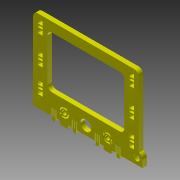
# Autodesk Inventor part: front
Saved by Autodesk Inventor 2012 SP1 (Build 160190100, 190)
## iProperties
Created: 2011-10-14
Part Number: front
Document SubType Name: Modeling
Designer: cramera
Density: 0.952 g/cm^3
Material: High Density Polyethylene
Mass: 331.479 g
Surface Area: 1014.12 cm^2
Volume: 348.192 cm^3
Autodesk Inventor part; units mm, degrees
ref_plane "YZ Plane" through (0, 0, 0) normal (1, 0, 0) x (0, 1, 0)
ref_plane "XZ Plane" through (0, 0, 0) normal (0, 1, 0) x (-1, 0, 0)
ref_plane "XY Plane" through (0, 0, 0) normal (0, 0, 1) x (1, 0, 0)
derived "skeleton.ipt"
sketch "DRILL-THROUGH" plane through (0, 0, 0) normal (0, 0, 1) x (1, 0, 0)
  arc A0 (646.0554, 82.7451) -> (647.6429, 84.3326) centre (646.0554, 84.3326) ccw
  arc A1 (646.0554, 116.9081) -> (644.4679, 115.3206) centre (646.0554, 115.3206) ccw
  arc A2 (644.4679, 115.3206) -> (646.0554, 113.7331) centre (646.0554, 115.3206) ccw
  arc A3 (646.0554, 113.7331) -> (647.6429, 115.3206) centre (646.0554, 115.3206) ccw
  arc A4 (647.6429, 115.3206) -> (646.0554, 116.9081) centre (646.0554, 115.3206) ccw
  arc A5 (677.0434, 116.9081) -> (675.4559, 115.3206) centre (677.0434, 115.3206) ccw
  arc A6 (675.4559, 115.3206) -> (677.0434, 113.7331) centre (677.0434, 115.3206) ccw
  arc A7 (677.0434, 113.7331) -> (678.6309, 115.3206) centre (677.0434, 115.3206) ccw
  arc A8 (678.6309, 115.3206) -> (677.0434, 116.9081) centre (677.0434, 115.3206) ccw
  arc A9 (646.0554, 85.9201) -> (644.4679, 84.3326) centre (646.0554, 84.3326) ccw
  arc A10 (644.4679, 84.3326) -> (646.0554, 82.7451) centre (646.0554, 84.3326) ccw
  arc A11 (647.6429, 84.3326) -> (646.0554, 85.9201) centre (646.0554, 84.3326) ccw
  arc A12 (677.0434, 85.9201) -> (675.4559, 84.3326) centre (677.0434, 84.3326) ccw
  arc A13 (675.4559, 84.3326) -> (677.0434, 82.7451) centre (677.0434, 84.3326) ccw
  arc A14 (677.0434, 82.7451) -> (678.6309, 84.3326) centre (677.0434, 84.3326) ccw
  arc A15 (678.6309, 84.3326) -> (677.0434, 85.9201) centre (677.0434, 84.3326) ccw
  constraints: 32 point on circle, 16 centre point
sketch "POCKET_1-16" plane through (0, 0, 0) normal (0, 0, 1) x (1, 0, 0)
  line L0 (766.5149, 230.5307) -> (766.5149, 224.7099)
  arc A0 (766.5149, 224.7099) -> (768.1024, 223.1224) centre (768.1024, 224.7099) ccw
  line L1 (768.1024, 223.1224) -> (774.717, 223.1224)
  arc A1 (774.717, 223.1224) -> (776.3045, 224.7099) centre (774.717, 224.7099) ccw
  line L2 (776.3045, 224.7099) -> (776.3045, 230.5307)
  arc A2 (776.3045, 230.5307) -> (774.717, 232.1182) centre (774.717, 230.5307) ccw
  arc A3 (776.3045, 238.6005) -> (771.4097, 243.4953) centre (771.4097, 238.6005) ccw
  arc A4 (771.4097, 243.4953) -> (766.5149, 238.6005) centre (771.4097, 238.6005) ccw
  arc A5 (766.5149, 238.6005) -> (771.4097, 233.7057) centre (771.4097, 238.6005) ccw
  arc A6 (771.4097, 233.7057) -> (776.3045, 238.6005) centre (771.4097, 238.6005) ccw
  line L3 (774.717, 232.1182) -> (768.1024, 232.1182)
  arc A7 (790.0628, 221.5349) -> (788.4753, 219.9474) centre (790.0628, 219.9474) ccw
  line L4 (788.4753, 219.9474) -> (788.4753, 213.3328)
  arc A8 (788.4753, 213.3328) -> (790.0628, 211.7453) centre (790.0628, 213.3328) ccw
  line L5 (790.0628, 211.7453) -> (796.6774, 211.7453)
  arc A9 (796.6774, 211.7453) -> (798.2649, 213.3328) centre (796.6774, 213.3328) ccw
  line L6 (798.2649, 213.3328) -> (798.2649, 219.9474)
  arc A10 (798.2649, 219.9474) -> (796.6774, 221.5349) centre (796.6774, 219.9474) ccw
  line L7 (796.6774, 221.5349) -> (790.0628, 221.5349)
  arc A11 (768.1024, 221.5349) -> (766.5149, 219.9474) centre (768.1024, 219.9474) ccw
  line L8 (766.5149, 219.9474) -> (766.5149, 213.3328)
  arc A12 (766.5149, 213.3328) -> (768.1024, 211.7453) centre (768.1024, 213.3328) ccw
  line L9 (768.1024, 211.7453) -> (774.717, 211.7453)
  arc A13 (774.717, 211.7453) -> (776.3045, 213.3328) centre (774.717, 213.3328) ccw
  line L10 (776.3045, 213.3328) -> (776.3045, 219.9474)
  arc A14 (776.3045, 219.9474) -> (774.717, 221.5349) centre (774.717, 219.9474) ccw
  line L11 (774.717, 221.5349) -> (768.1024, 221.5349)
  arc A15 (785.3003, 233.7057) -> (786.8878, 235.2932) centre (785.3003, 235.2932) ccw
  line L12 (786.8878, 235.2932) -> (786.8878, 241.9078)
  arc A16 (786.8878, 241.9078) -> (785.3003, 243.4953) centre (785.3003, 241.9078) ccw
  line L13 (785.3003, 243.4953) -> (779.4795, 243.4953)
  arc A17 (779.4795, 243.4953) -> (777.892, 241.9078) centre (779.4795, 241.9078) ccw
  line L14 (777.892, 241.9078) -> (777.892, 235.2932)
  arc A18 (777.892, 235.2932) -> (779.4795, 233.7057) centre (779.4795, 235.2932) ccw
  line L15 (779.4795, 233.7057) -> (785.3003, 233.7057)
  arc A19 (790.0628, 232.1182) -> (788.4753, 230.5307) centre (790.0628, 230.5307) ccw
  line L16 (788.4753, 230.5307) -> (788.4753, 224.7099)
  arc A20 (788.4753, 224.7099) -> (790.0628, 223.1224) centre (790.0628, 224.7099) ccw
  line L17 (790.0628, 223.1224) -> (796.6774, 223.1224)
  line L18 (798.2649, 224.7099) -> (798.2649, 230.5307)
  arc A21 (798.2649, 230.5307) -> (796.6774, 232.1182) centre (796.6774, 230.5307) ccw
  line L19 (796.6774, 232.1182) -> (790.0628, 232.1182)
  arc A22 (796.6774, 223.1224) -> (798.2649, 224.7099) centre (796.6774, 224.7099) ccw
  line L20 (777.892, 219.9474) -> (777.892, 213.3328)
  arc A23 (777.892, 213.3328) -> (779.4795, 211.7453) centre (779.4795, 213.3328) ccw
  line L21 (779.4795, 211.7453) -> (785.3003, 211.7453)
  arc A24 (785.3003, 211.7453) -> (786.8878, 213.3328) centre (785.3003, 213.3328) ccw
  line L22 (786.8878, 213.3328) -> (786.8878, 219.9474)
  arc A25 (786.8878, 219.9474) -> (785.3003, 221.5349) centre (785.3003, 219.9474) ccw
  line L23 (785.3003, 221.5349) -> (779.4795, 221.5349)
  arc A26 (786.8878, 227.6203) -> (782.3899, 232.1182) centre (782.3899, 227.6203) ccw
  arc A27 (782.3899, 232.1182) -> (777.892, 227.6203) centre (782.3899, 227.6203) ccw
  arc A28 (788.4753, 235.2932) -> (790.0628, 233.7057) centre (790.0628, 235.2932) ccw
  line L24 (790.0628, 233.7057) -> (796.6774, 233.7057)
  arc A29 (779.4795, 221.5349) -> (777.892, 219.9474) centre (779.4795, 219.9474) ccw
  arc A30 (768.1024, 232.1182) -> (766.5149, 230.5307) centre (768.1024, 230.5307) ccw
  arc A31 (777.892, 227.6203) -> (782.3899, 223.1224) centre (782.3899, 227.6203) ccw
  arc A32 (782.3899, 223.1224) -> (786.8878, 227.6203) centre (782.3899, 227.6203) ccw
  arc A33 (796.6774, 233.7057) -> (798.2649, 235.2932) centre (796.6774, 235.2932) ccw
  line L25 (798.2649, 235.2932) -> (798.2649, 241.9078)
  arc A34 (798.2649, 241.9078) -> (796.6774, 243.4953) centre (796.6774, 241.9078) ccw
  line L26 (796.6774, 243.4953) -> (790.0628, 243.4953)
  arc A35 (790.0628, 243.4953) -> (788.4753, 241.9078) centre (790.0628, 241.9078) ccw
  line L27 (788.4753, 241.9078) -> (788.4753, 235.2932)
  constraints: 72 point on circle, 56 end point, 36 centre point
sketch "POCKET_3-8" plane through (0, 0, 0) normal (0, 0, 1) x (1, 0, 0)
  circle A0 centre (796.1694, 92.6193) radius 12.7
  constraints: 1 centre point
sketch "STOCK_12MM" plane through (0, 0, 0) normal (0, 0, 1) x (1, 0, 0)
  line L0 (457.2, 0) -> (914.4, 0)
  line L1 (914.4, 0) -> (914.4, 914.4)
  line L2 (914.4, 914.4) -> (457.2, 914.4)
  line L3 (457.2, 914.4) -> (457.2, 0)
  line L4 (457.2, 0) -> (457.2, 914.4)
  constraints: 10 end point
sketch "THROUGH-CUT" plane through (0, 0, 0) normal (0, 0, 1) x (1, 0, 0)
  line L0 (546.8684, 124.1379) -> (546.8684, 124.7278)
  arc A0 (546.8684, 124.7278) -> (546.8684, 126.9728) centre (545.7459, 125.8503) ccw
  arc A1 (546.8684, 126.9728) -> (544.6234, 126.9728) centre (545.7459, 125.8503) ccw
  line L1 (544.6234, 126.9728) -> (536.7945, 126.9728)
  circle A2 centre (604.3994, 99.8266) radius 5.925
  circle A3 centre (718.6994, 99.8266) radius 5.925
  circle A4 centre (796.1694, 92.6193) radius 7.3025
  circle A5 centre (661.5494, 99.8266) radius 14.2875
  line L2 (534.5494, 116.3458) -> (534.5494, 110.6759)
  arc A6 (534.5494, 110.6759) -> (534.5494, 108.4308) centre (535.6719, 109.5534) ccw
  arc A7 (534.5494, 108.4308) -> (536.7945, 108.4308) centre (535.6719, 109.5534) ccw
  line L3 (536.7945, 108.4308) -> (544.6234, 108.4308)
  arc A8 (544.6234, 108.4308) -> (546.8684, 110.6759) centre (545.7459, 109.5534) ccw
  line L4 (546.8684, 110.6759) -> (546.8684, 116.3458)
  arc A9 (546.8684, 116.3458) -> (546.8684, 118.5908) centre (545.7459, 117.4683) ccw
  arc A10 (546.8684, 118.5908) -> (544.6234, 118.5908) centre (545.7459, 117.4683) ccw
  line L5 (544.6234, 118.5908) -> (536.7945, 118.5908)
  arc A11 (536.7945, 118.5908) -> (534.5494, 116.3458) centre (535.6719, 117.4683) ccw
  line L6 (536.7945, 130.2748) -> (544.6234, 130.2748)
  arc A12 (544.6234, 130.2748) -> (546.8684, 130.2748) centre (545.7459, 131.3974) ccw
  arc A13 (546.8684, 130.2748) -> (546.8684, 132.5199) centre (545.7459, 131.3974) ccw
  line L7 (546.8684, 132.5199) -> (546.8684, 138.1898)
  arc A14 (546.8684, 138.1898) -> (546.8684, 140.4348) centre (545.7459, 139.3123) ccw
  arc A15 (546.8684, 140.4348) -> (544.6234, 140.4348) centre (545.7459, 139.3123) ccw
  line L8 (544.6234, 140.4348) -> (536.7945, 140.4348)
  arc A16 (536.7945, 140.4348) -> (534.5494, 138.1898) centre (535.6719, 139.3123) ccw
  line L9 (534.5494, 138.1898) -> (534.5494, 132.5199)
  arc A17 (534.5494, 132.5199) -> (536.7945, 130.2748) centre (535.6719, 131.3974) ccw
  line L10 (534.5494, 256.0458) -> (534.5494, 250.3759)
  arc A18 (534.5494, 250.3759) -> (534.5494, 248.1308) centre (535.6719, 249.2534) ccw
  arc A19 (534.5494, 248.1308) -> (536.7945, 248.1308) centre (535.6719, 249.2534) ccw
  line L11 (536.7945, 248.1308) -> (544.6234, 248.1308)
  arc A20 (544.6234, 248.1308) -> (546.8684, 248.1308) centre (545.7459, 249.2534) ccw
  arc A21 (546.8684, 248.1308) -> (546.8684, 250.3759) centre (545.7459, 249.2534) ccw
  line L12 (546.8684, 250.3759) -> (546.8684, 256.0458)
  arc A22 (546.8684, 256.0458) -> (546.8684, 258.2908) centre (545.7459, 257.1683) ccw
  arc A23 (546.8684, 258.2908) -> (544.6234, 258.2908) centre (545.7459, 257.1683) ccw
  line L13 (544.6234, 258.2908) -> (536.7945, 258.2908)
  arc A24 (536.7945, 258.2908) -> (534.5494, 258.2908) centre (535.6719, 257.1683) ccw
  arc A25 (534.5494, 258.2908) -> (534.5494, 256.0458) centre (535.6719, 257.1683) ccw
  arc A26 (786.3044, 248.1308) -> (788.5494, 250.3759) centre (787.4269, 249.2534) ccw
  line L14 (788.5494, 250.3759) -> (788.5494, 256.0458)
  arc A27 (788.5494, 256.0458) -> (786.3044, 258.2908) centre (787.4269, 257.1683) ccw
  line L15 (786.3044, 258.2908) -> (778.4755, 258.2908)
  arc A28 (778.4755, 258.2908) -> (776.2304, 256.0458) centre (777.3529, 257.1683) ccw
  line L16 (776.2304, 256.0458) -> (776.2304, 250.3759)
  arc A29 (776.2304, 250.3759) -> (778.4755, 248.1308) centre (777.3529, 249.2534) ccw
  line L17 (778.4755, 248.1308) -> (786.3044, 248.1308)
  arc A30 (786.3044, 269.9748) -> (788.5494, 272.2199) centre (787.4269, 271.0974) ccw
  line L18 (788.5494, 272.2199) -> (788.5494, 277.8898)
  arc A31 (788.5494, 277.8898) -> (786.3044, 280.1348) centre (787.4269, 279.0123) ccw
  line L19 (786.3044, 280.1348) -> (778.4755, 280.1348)
  arc A32 (778.4755, 280.1348) -> (776.2304, 277.8898) centre (777.3529, 279.0123) ccw
  line L20 (776.2304, 277.8898) -> (776.2304, 272.2199)
  arc A33 (776.2304, 272.2199) -> (778.4755, 269.9748) centre (777.3529, 271.0974) ccw
  line L21 (778.4755, 269.9748) -> (786.3044, 269.9748)
  arc A34 (536.7945, 193.6478) -> (534.5494, 191.4028) centre (535.6719, 192.5253) ccw
  line L22 (534.5494, 191.4028) -> (534.5494, 190.8129)
  arc A35 (534.5494, 190.8129) -> (536.7945, 188.5678) centre (535.6719, 189.6904) ccw
  line L23 (536.7945, 188.5678) -> (544.6234, 188.5678)
  arc A36 (544.6234, 188.5678) -> (546.8684, 188.5678) centre (545.7459, 189.6904) ccw
  arc A37 (546.8684, 188.5678) -> (546.8684, 190.8129) centre (545.7459, 189.6904) ccw
  line L24 (546.8684, 190.8129) -> (546.8684, 191.4028)
  arc A38 (546.8684, 191.4028) -> (546.8684, 193.6478) centre (545.7459, 192.5253) ccw
  arc A39 (546.8684, 193.6478) -> (544.6234, 193.6478) centre (545.7459, 192.5253) ccw
  line L25 (544.6234, 193.6478) -> (536.7945, 193.6478)
  arc A40 (786.3044, 261.5928) -> (788.5494, 263.8379) centre (787.4269, 262.7154) ccw
  line L26 (788.5494, 263.8379) -> (788.5494, 264.4278)
  arc A41 (788.5494, 264.4278) -> (786.3044, 266.6728) centre (787.4269, 265.5503) ccw
  line L27 (786.3044, 266.6728) -> (778.4755, 266.6728)
  arc A42 (778.4755, 266.6728) -> (776.2304, 264.4278) centre (777.3529, 265.5503) ccw
  line L28 (776.2304, 264.4278) -> (776.2304, 263.8379)
  arc A43 (776.2304, 263.8379) -> (778.4755, 261.5928) centre (777.3529, 262.7154) ccw
  line L29 (778.4755, 261.5928) -> (786.3044, 261.5928)
  line L30 (534.5494, 204.8648) -> (534.5494, 199.1949)
  arc A44 (534.5494, 199.1949) -> (534.5494, 196.9498) centre (535.6719, 198.0724) ccw
  arc A45 (534.5494, 196.9498) -> (536.7945, 196.9498) centre (535.6719, 198.0724) ccw
  line L31 (536.7945, 196.9498) -> (544.6234, 196.9498)
  arc A46 (544.6234, 196.9498) -> (546.8684, 196.9498) centre (545.7459, 198.0724) ccw
  arc A47 (546.8684, 196.9498) -> (546.8684, 199.1949) centre (545.7459, 198.0724) ccw
  line L32 (546.8684, 199.1949) -> (546.8684, 204.8648)
  arc A48 (546.8684, 204.8648) -> (546.8684, 207.1098) centre (545.7459, 205.9873) ccw
  arc A49 (546.8684, 207.1098) -> (544.6234, 207.1098) centre (545.7459, 205.9873) ccw
  line L33 (544.6234, 207.1098) -> (536.7945, 207.1098)
  arc A50 (536.7945, 207.1098) -> (534.5494, 204.8648) centre (535.6719, 205.9873) ccw
  line L34 (534.5494, 183.0208) -> (534.5494, 177.3509)
  arc A51 (534.5494, 177.3509) -> (534.5494, 175.1058) centre (535.6719, 176.2284) ccw
  arc A52 (534.5494, 175.1058) -> (536.7945, 175.1058) centre (535.6719, 176.2284) ccw
  line L35 (536.7945, 175.1058) -> (544.6234, 175.1058)
  arc A53 (544.6234, 175.1058) -> (546.8684, 177.3509) centre (545.7459, 176.2284) ccw
  line L36 (546.8684, 177.3509) -> (546.8684, 183.0208)
  arc A54 (546.8684, 183.0208) -> (546.8684, 185.2658) centre (545.7459, 184.1433) ccw
  arc A55 (546.8684, 185.2658) -> (544.6234, 185.2658) centre (545.7459, 184.1433) ccw
  line L37 (544.6234, 185.2658) -> (536.7945, 185.2658)
  arc A56 (536.7945, 185.2658) -> (534.5494, 183.0208) centre (535.6719, 184.1433) ccw
  arc A57 (786.3044, 175.1058) -> (788.5494, 177.3509) centre (787.4269, 176.2284) ccw
  line L38 (788.5494, 177.3509) -> (788.5494, 183.0208)
  arc A58 (788.5494, 183.0208) -> (786.3044, 185.2658) centre (787.4269, 184.1433) ccw
  line L39 (786.3044, 185.2658) -> (778.4755, 185.2658)
  arc A59 (778.4755, 185.2658) -> (776.2304, 183.0208) centre (777.3529, 184.1433) ccw
  arc A60 (776.2304, 177.3509) -> (778.4755, 175.1058) centre (777.3529, 176.2284) ccw
  line L40 (778.4755, 175.1058) -> (786.3044, 175.1058)
  arc A61 (786.3044, 188.5678) -> (788.5494, 190.8129) centre (787.4269, 189.6904) ccw
  line L41 (788.5494, 190.8129) -> (788.5494, 191.4028)
  arc A62 (788.5494, 191.4028) -> (786.3044, 193.6478) centre (787.4269, 192.5253) ccw
  line L42 (786.3044, 193.6478) -> (778.4755, 193.6478)
  arc A63 (778.4755, 193.6478) -> (776.2304, 191.4028) centre (777.3529, 192.5253) ccw
  line L43 (776.2304, 191.4028) -> (776.2304, 190.8129)
  arc A64 (776.2304, 190.8129) -> (778.4755, 188.5678) centre (777.3529, 189.6904) ccw
  line L44 (778.4755, 188.5678) -> (786.3044, 188.5678)
  arc A65 (786.3044, 121.8928) -> (788.5494, 124.1379) centre (787.4269, 123.0154) ccw
  line L45 (788.5494, 124.1379) -> (788.5494, 124.7278)
  arc A66 (788.5494, 124.7278) -> (786.3044, 126.9728) centre (787.4269, 125.8503) ccw
  line L46 (786.3044, 126.9728) -> (778.4755, 126.9728)
  arc A67 (778.4755, 126.9728) -> (776.2304, 124.7278) centre (777.3529, 125.8503) ccw
  line L47 (776.2304, 124.7278) -> (776.2304, 124.1379)
  arc A68 (776.2304, 124.1379) -> (778.4755, 121.8928) centre (777.3529, 123.0154) ccw
  line L48 (778.4755, 121.8928) -> (786.3044, 121.8928)
  arc A69 (786.3044, 130.2748) -> (788.5494, 132.5199) centre (787.4269, 131.3974) ccw
  line L49 (788.5494, 132.5199) -> (788.5494, 138.1898)
  arc A70 (788.5494, 138.1898) -> (786.3044, 140.4348) centre (787.4269, 139.3123) ccw
  line L50 (786.3044, 140.4348) -> (778.4755, 140.4348)
  arc A71 (778.4755, 140.4348) -> (776.2304, 138.1898) centre (777.3529, 139.3123) ccw
  line L51 (776.2304, 138.1898) -> (776.2304, 132.5199)
  arc A72 (776.2304, 132.5199) -> (778.4755, 130.2748) centre (777.3529, 131.3974) ccw
  line L52 (778.4755, 130.2748) -> (786.3044, 130.2748)
  line L53 (536.7945, 269.9748) -> (544.6234, 269.9748)
  arc A73 (544.6234, 269.9748) -> (546.8684, 269.9748) centre (545.7459, 271.0974) ccw
  arc A74 (546.8684, 269.9748) -> (546.8684, 272.2199) centre (545.7459, 271.0974) ccw
  line L54 (546.8684, 272.2199) -> (546.8684, 277.8898)
  arc A75 (546.8684, 277.8898) -> (546.8684, 280.1348) centre (545.7459, 279.0123) ccw
  arc A76 (546.8684, 280.1348) -> (544.6234, 280.1348) centre (545.7459, 279.0123) ccw
  line L55 (544.6234, 280.1348) -> (536.7945, 280.1348)
  arc A77 (536.7945, 280.1348) -> (534.5494, 277.8898) centre (535.6719, 279.0123) ccw
  line L56 (534.5494, 277.8898) -> (534.5494, 272.2199)
  arc A78 (534.5494, 272.2199) -> (536.7945, 269.9748) centre (535.6719, 271.0974) ccw
  line L57 (776.2304, 183.0208) -> (776.2304, 177.3509)
  arc A79 (536.7945, 126.9728) -> (534.5494, 124.7278) centre (535.6719, 125.8503) ccw
  arc A80 (786.3044, 196.9498) -> (788.5494, 199.1949) centre (787.4269, 198.0724) ccw
  line L58 (788.5494, 199.1949) -> (788.5494, 204.8648)
  arc A81 (788.5494, 204.8648) -> (786.3044, 207.1098) centre (787.4269, 205.9873) ccw
  line L59 (786.3044, 207.1098) -> (778.4755, 207.1098)
  arc A82 (778.4755, 207.1098) -> (776.2304, 204.8648) centre (777.3529, 205.9873) ccw
  line L60 (776.2304, 204.8648) -> (776.2304, 199.1949)
  arc A83 (776.2304, 199.1949) -> (778.4755, 196.9498) centre (777.3529, 198.0724) ccw
  line L61 (778.4755, 196.9498) -> (786.3044, 196.9498)
  arc A84 (776.2304, 110.6759) -> (778.4755, 108.4308) centre (777.3529, 109.5534) ccw
  line L62 (778.4755, 108.4308) -> (786.3044, 108.4308)
  arc A85 (786.3044, 108.4308) -> (788.5494, 110.6759) centre (787.4269, 109.5534) ccw
  line L63 (788.5494, 110.6759) -> (788.5494, 116.3458)
  arc A86 (788.5494, 116.3458) -> (786.3044, 118.5908) centre (787.4269, 117.4683) ccw
  line L64 (786.3044, 118.5908) -> (778.4755, 118.5908)
  arc A87 (778.4755, 118.5908) -> (776.2304, 116.3458) centre (777.3529, 117.4683) ccw
  line L65 (776.2304, 116.3458) -> (776.2304, 110.6759)
  arc A88 (534.5494, 263.8379) -> (536.7945, 261.5928) centre (535.6719, 262.7154) ccw
  line L66 (536.7945, 261.5928) -> (544.6234, 261.5928)
  arc A89 (544.6234, 261.5928) -> (546.8684, 261.5928) centre (545.7459, 262.7154) ccw
  arc A90 (546.8684, 261.5928) -> (546.8684, 263.8379) centre (545.7459, 262.7154) ccw
  line L67 (546.8684, 263.8379) -> (546.8684, 264.4278)
  arc A91 (546.8684, 264.4278) -> (546.8684, 266.6728) centre (545.7459, 265.5503) ccw
  arc A92 (546.8684, 266.6728) -> (544.6234, 266.6728) centre (545.7459, 265.5503) ccw
  line L68 (544.6234, 266.6728) -> (536.7945, 266.6728)
  arc A93 (536.7945, 266.6728) -> (534.5494, 264.4278) centre (535.6719, 265.5503) ccw
  line L69 (534.5494, 264.4278) -> (534.5494, 263.8379)
  line L70 (559.9494, 254.6078) -> (559.9494, 143.4828)
  arc A94 (559.9494, 143.4828) -> (572.6494, 130.7828) centre (572.6494, 143.4828) ccw
  line L71 (572.6494, 130.7828) -> (750.4494, 130.7828)
  arc A95 (750.4494, 130.7828) -> (763.1494, 143.4828) centre (750.4494, 143.4828) ccw
  line L72 (763.1494, 143.4828) -> (763.1494, 254.6078)
  arc A96 (763.1494, 254.6078) -> (750.4494, 267.3078) centre (750.4494, 254.6078) ccw
  line L73 (750.4494, 267.3078) -> (572.6494, 267.3078)
  arc A97 (572.6494, 267.3078) -> (559.9494, 254.6078) centre (572.6494, 254.6078) ccw
  line L74 (534.5494, 124.7278) -> (534.5494, 124.1379)
  arc A98 (534.5494, 124.1379) -> (536.7945, 121.8928) centre (535.6719, 123.0154) ccw
  line L75 (536.7945, 121.8928) -> (544.6234, 121.8928)
  arc A99 (544.6234, 121.8928) -> (546.8684, 121.8928) centre (545.7459, 123.0154) ccw
  arc A100 (546.8684, 121.8928) -> (546.8684, 124.1379) centre (545.7459, 123.0154) ccw
  arc A101 (691.8887, 77.9794) -> (693.4762, 79.5669) centre (691.8887, 79.5669) ccw
  line L76 (691.8887, 77.9794) -> (691.7617, 77.9794)
  arc A102 (690.1742, 79.5669) -> (691.7617, 77.9794) centre (691.7617, 79.5669) ccw
  line L77 (690.1742, 79.5669) -> (690.1742, 94.2703)
  arc A103 (691.7617, 95.8578) -> (690.1742, 94.2703) centre (691.7617, 94.2703) ccw
  line L78 (691.7617, 95.8578) -> (691.8887, 95.8578)
  arc A104 (693.4762, 94.2703) -> (691.8887, 95.8578) centre (691.8887, 94.2703) ccw
  line L79 (693.4762, 94.2703) -> (693.4762, 79.5669)
  arc A105 (575.3936, 79.5669) -> (576.9811, 77.9794) centre (576.9811, 79.5669) ccw
  line L80 (575.3936, 79.5669) -> (575.3936, 94.2703)
  arc A106 (576.9811, 95.8578) -> (575.3936, 94.2703) centre (576.9811, 94.2703) ccw
  line L81 (576.9811, 95.8578) -> (577.1081, 95.8578)
  arc A107 (578.6956, 94.2703) -> (577.1081, 95.8578) centre (577.1081, 94.2703) ccw
  line L82 (578.6956, 94.2703) -> (578.6956, 79.5669)
  arc A108 (577.1081, 77.9794) -> (578.6956, 79.5669) centre (577.1081, 79.5669) ccw
  line L83 (577.1081, 77.9794) -> (576.9811, 77.9794)
  arc A109 (631.3371, 77.9794) -> (632.9246, 79.5669) centre (631.3371, 79.5669) ccw
  line L84 (632.9246, 79.5669) -> (632.9246, 94.2703)
  arc A110 (632.9246, 94.2703) -> (631.3371, 95.8578) centre (631.3371, 94.2703) ccw
  line L85 (631.3371, 95.8578) -> (631.2101, 95.8578)
  arc A111 (631.2101, 95.8578) -> (629.6226, 94.2703) centre (631.2101, 94.2703) ccw
  line L86 (629.6226, 94.2703) -> (629.6226, 79.5669)
  arc A112 (629.6226, 79.5669) -> (631.2101, 77.9794) centre (631.2101, 79.5669) ccw
  line L87 (631.2101, 77.9794) -> (631.3371, 77.9794)
  arc A113 (744.4032, 79.5669) -> (745.9907, 77.9794) centre (745.9907, 79.5669) ccw
  line L88 (745.9907, 77.9794) -> (746.1177, 77.9794)
  arc A114 (746.1177, 77.9794) -> (747.7052, 79.5669) centre (746.1177, 79.5669) ccw
  line L89 (747.7052, 79.5669) -> (747.7052, 94.2703)
  arc A115 (747.7052, 94.2703) -> (746.1177, 95.8578) centre (746.1177, 94.2703) ccw
  line L90 (746.1177, 95.8578) -> (745.9907, 95.8578)
  arc A116 (745.9907, 95.8578) -> (744.4032, 94.2703) centre (745.9907, 94.2703) ccw
  line L91 (744.4032, 94.2703) -> (744.4032, 79.5669)
  arc A117 (723.6352, 87.8143) -> (725.8803, 87.8143) centre (724.7577, 88.9369) ccw
  line L92 (723.6352, 87.8143) -> (722.9636, 88.486)
  arc A118 (707.3588, 104.0907) -> (722.9636, 88.486) centre (718.6994, 99.8266) ccw
  line L93 (707.3588, 104.0907) -> (706.6872, 104.7624)
  arc A119 (706.6872, 107.0074) -> (706.6872, 104.7624) centre (707.8097, 105.8849) ccw
  line L94 (706.6872, 107.0074) -> (706.759, 107.0793)
  arc A120 (709.0041, 107.0793) -> (706.759, 107.0793) centre (707.8816, 105.9567) ccw
  line L95 (709.0041, 107.0793) -> (710.4878, 105.5956)
  arc A121 (710.7864, 103.7656) -> (710.4878, 105.5956) centre (709.3653, 104.473) ccw
  arc A122 (710.7864, 103.7656) -> (722.6384, 91.9136) centre (718.6994, 99.8266) ccw
  arc A123 (724.4684, 91.615) -> (722.6384, 91.9136) centre (723.3459, 90.4924) ccw
  line L96 (724.4684, 91.615) -> (725.9521, 90.1312)
  arc A124 (725.9521, 87.8862) -> (725.9521, 90.1312) centre (724.8296, 89.0087) ccw
  line L97 (725.9521, 87.8862) -> (725.8803, 87.8143)
  arc A125 (713.7636, 111.8388) -> (711.5186, 111.8388) centre (712.6411, 110.7163) ccw
  line L98 (713.7636, 111.8388) -> (714.4352, 111.1672)
  arc A126 (730.04, 95.5624) -> (714.4352, 111.1672) centre (718.6994, 99.8266) ccw
  line L99 (730.04, 95.5624) -> (730.7117, 94.8908)
  arc A127 (730.7117, 92.6457) -> (730.7117, 94.8908) centre (729.5891, 93.7682) ccw
  line L100 (730.7117, 92.6457) -> (730.6398, 92.5739)
  arc A128 (728.3947, 92.5739) -> (730.6398, 92.5739) centre (729.5173, 93.6964) ccw
  line L101 (728.3947, 92.5739) -> (726.911, 94.0576)
  arc A129 (726.6124, 95.8876) -> (726.911, 94.0576) centre (728.0336, 95.1801) ccw
  arc A130 (726.6124, 95.8876) -> (714.7604, 107.7396) centre (718.6994, 99.8266) ccw
  arc A131 (712.9304, 108.0382) -> (714.7604, 107.7396) centre (714.053, 109.1607) ccw
  line L102 (712.9304, 108.0382) -> (711.4467, 109.5219)
  arc A132 (711.4467, 111.767) -> (711.4467, 109.5219) centre (712.5692, 110.6444) ccw
  line L103 (711.4467, 111.767) -> (711.5186, 111.8388)
  arc A133 (592.459, 92.5739) -> (594.7041, 92.5739) centre (593.5816, 93.6964) ccw
  line L104 (592.459, 92.5739) -> (592.3872, 92.6457)
  arc A134 (592.3872, 94.8908) -> (592.3872, 92.6457) centre (593.5097, 93.7682) ccw
  line L105 (592.3872, 94.8908) -> (593.0588, 95.5624)
  arc A135 (608.6636, 111.1672) -> (593.0588, 95.5624) centre (604.3994, 99.8266) ccw
  line L106 (608.6636, 111.1672) -> (609.3352, 111.8388)
  arc A136 (611.5803, 111.8388) -> (609.3352, 111.8388) centre (610.4577, 110.7163) ccw
  line L107 (611.5803, 111.8388) -> (611.6521, 111.767)
  arc A137 (611.6521, 109.5219) -> (611.6521, 111.767) centre (610.5296, 110.6444) ccw
  line L108 (611.6521, 109.5219) -> (610.1684, 108.0382)
  arc A138 (608.3384, 107.7396) -> (610.1684, 108.0382) centre (609.0459, 109.1607) ccw
  arc A139 (608.3384, 107.7396) -> (596.4864, 95.8876) centre (604.3994, 99.8266) ccw
  arc A140 (596.1878, 94.0576) -> (596.4864, 95.8876) centre (595.0653, 95.1801) ccw
  line L109 (596.1878, 94.0576) -> (594.7041, 92.5739)
  line L110 (753.0392, 94.2703) -> (753.0392, 76.8078)
  line L111 (753.0392, 76.8078) -> (810.7744, 76.8078)
  line L112 (810.7744, 76.8078) -> (810.7744, 94.2068)
  arc A141 (810.7744, 94.2068) -> (802.1832, 107.5162) centre (796.1694, 94.2068) ccw
  arc A142 (801.2494, 108.9629) -> (802.1832, 107.5162) centre (802.8369, 108.9629) ccw
  line L113 (801.2494, 108.9629) -> (801.2494, 280.0078)
  arc A143 (801.2494, 280.0078) -> (788.5494, 292.7078) centre (788.5494, 280.0078) ccw
  line L114 (788.5494, 292.7078) -> (534.5494, 292.7078)
  arc A144 (534.5494, 292.7078) -> (521.8494, 280.0078) centre (534.5494, 280.0078) ccw
  line L115 (521.8494, 280.0078) -> (521.8494, 76.8078)
  line L116 (521.8494, 76.8078) -> (570.0596, 76.8078)
  line L117 (570.0596, 76.8078) -> (570.0596, 94.2703)
  arc A145 (571.6471, 95.8578) -> (570.0596, 94.2703) centre (571.6471, 94.2703) ccw
  line L118 (571.6471, 95.8578) -> (571.7741, 95.8578)
  arc A146 (573.3616, 94.2703) -> (571.7741, 95.8578) centre (571.7741, 94.2703) ccw
  line L119 (573.3616, 94.2703) -> (573.3616, 74.3551)
  line L120 (573.3616, 74.3551) -> (573.3616, 71.7278)
  line L121 (573.3616, 71.7278) -> (571.8376, 70.4578)
  line L122 (571.8376, 70.4578) -> (571.8376, 68.7399)
  line L123 (571.8376, 68.7399) -> (575.4372, 67.9178)
  line L124 (575.4372, 67.9178) -> (579.1423, 67.9178)
  arc A147 (579.1423, 67.9178) -> (580.7276, 69.5053) centre (579.1401, 69.5053) ccw
  line L125 (580.7276, 69.5053) -> (580.7276, 94.2703)
  arc A148 (582.3151, 95.8578) -> (580.7276, 94.2703) centre (582.3151, 94.2703) ccw
  line L126 (582.3151, 95.8578) -> (582.4421, 95.8578)
  arc A149 (584.0296, 94.2703) -> (582.4421, 95.8578) centre (582.4421, 94.2703) ccw
  line L127 (584.0296, 94.2703) -> (584.0296, 76.8078)
  line L128 (584.0296, 76.8078) -> (591.4365, 76.8078)
  arc A150 (593.6816, 74.5628) -> (591.4365, 76.8078) centre (592.5591, 75.6853) ccw
  line L129 (593.6816, 74.5628) -> (593.6816, 69.5053)
  line L130 (593.6816, 69.5053) -> (595.2691, 67.9178)
  line L131 (595.2691, 67.9178) -> (613.0491, 67.9178)
  line L132 (613.0491, 67.9178) -> (614.6366, 69.5053)
  line L133 (614.6366, 69.5053) -> (614.6366, 74.5628)
  arc A151 (616.8817, 76.8078) -> (614.6366, 74.5628) centre (615.7591, 75.6853) ccw
  line L134 (616.8817, 76.8078) -> (624.2886, 76.8078)
  line L135 (624.2886, 76.8078) -> (624.2886, 94.2703)
  arc A152 (625.8761, 95.8578) -> (624.2886, 94.2703) centre (625.8761, 94.2703) ccw
  line L136 (625.8761, 95.8578) -> (626.0031, 95.8578)
  arc A153 (627.5906, 94.2703) -> (626.0031, 95.8578) centre (626.0031, 94.2703) ccw
  line L137 (627.5906, 94.2703) -> (627.5906, 69.5053)
  arc A154 (627.5906, 69.5053) -> (629.1781, 67.9178) centre (629.1781, 69.5053) ccw
  line L138 (629.1781, 67.9178) -> (632.881, 67.9178)
  line L139 (632.881, 67.9178) -> (636.4806, 68.7399)
  line L140 (636.4806, 68.7399) -> (636.4806, 70.4578)
  line L141 (636.4806, 70.4578) -> (634.9566, 71.7278)
  line L142 (634.9566, 71.7278) -> (634.9566, 74.3551)
  line L143 (634.9566, 74.3551) -> (634.9566, 94.2703)
  arc A155 (636.5441, 95.8578) -> (634.9566, 94.2703) centre (636.5441, 94.2703) ccw
  line L144 (636.5441, 95.8578) -> (636.6711, 95.8578)
  arc A156 (638.2586, 94.2703) -> (636.6711, 95.8578) centre (636.6711, 94.2703) ccw
  line L145 (638.2586, 94.2703) -> (638.2586, 76.8078)
  line L146 (638.2586, 76.8078) -> (684.8402, 76.8078)
  line L147 (684.8402, 76.8078) -> (684.8402, 94.2703)
  arc A157 (686.4277, 95.8578) -> (684.8402, 94.2703) centre (686.4277, 94.2703) ccw
  line L148 (686.4277, 95.8578) -> (686.5547, 95.8578)
  arc A158 (688.1422, 94.2703) -> (686.5547, 95.8578) centre (686.5547, 94.2703) ccw
  line L149 (688.1422, 94.2703) -> (688.1422, 74.3551)
  line L150 (688.1422, 74.3551) -> (688.1422, 71.7278)
  line L151 (688.1422, 71.7278) -> (686.6182, 70.4578)
  line L152 (686.6182, 70.4578) -> (686.6182, 68.7399)
  line L153 (686.6182, 68.7399) -> (690.2178, 67.9178)
  line L154 (690.2178, 67.9178) -> (693.9207, 67.9178)
  arc A159 (693.9207, 67.9178) -> (695.5082, 69.5053) centre (693.9207, 69.5053) ccw
  line L155 (695.5082, 69.5053) -> (695.5082, 94.2703)
  arc A160 (697.0957, 95.8578) -> (695.5082, 94.2703) centre (697.0957, 94.2703) ccw
  line L156 (697.0957, 95.8578) -> (697.2227, 95.8578)
  arc A161 (698.8102, 94.2703) -> (697.2227, 95.8578) centre (697.2227, 94.2703) ccw
  line L157 (698.8102, 94.2703) -> (698.8102, 76.8078)
  line L158 (698.8102, 76.8078) -> (706.2172, 76.8078)
  arc A162 (708.4622, 74.5628) -> (706.2172, 76.8078) centre (707.3397, 75.6853) ccw
  line L159 (708.4622, 74.5628) -> (708.4622, 69.5053)
  line L160 (708.4622, 69.5053) -> (710.0497, 67.9178)
  line L161 (710.0497, 67.9178) -> (727.8297, 67.9178)
  line L162 (727.8297, 67.9178) -> (729.4172, 69.5053)
  line L163 (729.4172, 69.5053) -> (729.4172, 74.5628)
  arc A163 (731.6623, 76.8078) -> (729.4172, 74.5628) centre (730.5398, 75.6853) ccw
  line L164 (731.6623, 76.8078) -> (739.0692, 76.8078)
  line L165 (739.0692, 76.8078) -> (739.0692, 94.2703)
  arc A164 (740.6567, 95.8578) -> (739.0692, 94.2703) centre (740.6567, 94.2703) ccw
  line L166 (740.6567, 95.8578) -> (740.7837, 95.8578)
  arc A165 (742.3712, 94.2703) -> (740.7837, 95.8578) centre (740.7837, 94.2703) ccw
  line L167 (742.3712, 94.2703) -> (742.3712, 69.5053)
  arc A166 (742.3712, 69.5053) -> (743.9566, 67.9178) centre (743.9587, 69.5053) ccw
  line L168 (743.9566, 67.9178) -> (747.6617, 67.9178)
  line L169 (747.6617, 67.9178) -> (751.2612, 68.7399)
  line L170 (751.2612, 68.7399) -> (751.2612, 70.4578)
  line L171 (751.2612, 70.4578) -> (749.7372, 71.7278)
  line L172 (749.7372, 71.7278) -> (749.7372, 74.3551)
  line L173 (749.7372, 74.3551) -> (749.7372, 94.2703)
  arc A167 (751.3247, 95.8578) -> (749.7372, 94.2703) centre (751.3247, 94.2703) ccw
  line L174 (751.3247, 95.8578) -> (751.4517, 95.8578)
  arc A168 (753.0392, 94.2703) -> (751.4517, 95.8578) centre (751.4517, 94.2703) ccw
  arc A169 (600.1352, 88.486) -> (615.74, 104.0907) centre (604.3994, 99.8266) ccw
  line L175 (600.1352, 88.486) -> (599.4636, 87.8143)
  arc A170 (597.2186, 87.8143) -> (599.4636, 87.8143) centre (598.3411, 88.9369) ccw
  line L176 (597.2186, 87.8143) -> (597.1467, 87.8862)
  arc A171 (597.1467, 90.1312) -> (597.1467, 87.8862) centre (598.2692, 89.0087) ccw
  line L177 (597.1467, 90.1312) -> (598.6304, 91.615)
  arc A172 (600.4604, 91.9136) -> (598.6304, 91.615) centre (599.753, 90.4924) ccw
  arc A173 (600.4604, 91.9136) -> (612.3124, 103.7656) centre (604.3994, 99.8266) ccw
  arc A174 (612.611, 105.5956) -> (612.3124, 103.7656) centre (613.7336, 104.473) ccw
  line L178 (612.611, 105.5956) -> (614.0947, 107.0793)
  arc A175 (616.3398, 107.0793) -> (614.0947, 107.0793) centre (615.2173, 105.9567) ccw
  line L179 (616.3398, 107.0793) -> (616.4117, 107.0074)
  arc A176 (616.4117, 104.7624) -> (616.4117, 107.0074) centre (615.2891, 105.8849) ccw
  line L180 (616.4117, 104.7624) -> (615.74, 104.0907)
  dimension "d7" = 11.85
  dimension "d8" = 11.85
  constraints: 362 end point, 346 point on circle, 177 centre point
  measures "d7" diameter of A2
  measures "d8" diameter of A3
extrude "Extrusion1" add sketch "THROUGH-CUT" along normal blind 12
extrude "Extrusion2" cut sketch "POCKET_3-8" along normal blind 9.525
extrude "Extrusion3" cut sketch "POCKET_1-16" along normal blind 1.5875
equation "\"d8\" = d7"
equation "\"d1\" = StockThickness"
equation "\"StockThickness\" = 12"
body "Solid1"
